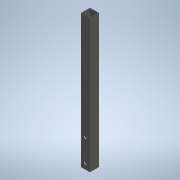
# Autodesk Inventor part: Carbon Fiber Arm
Saved by Autodesk Inventor 2021 (Build 250183000, 183)
## iProperties
Created: 2020-04-12
Part Number: Carbon Fiber Arm
Material: Generic
Document SubType Name: Modeling
Designer: chutsu
Density: 1 g/cm^3
Appearance: Default
Author: chutsu
Autodesk Inventor part; units mm, degrees
ref_plane "YZ Plane" through (0, 0, 0) normal (1, 0, 0) x (0, 1, 0)
ref_plane "XZ Plane" through (0, 0, 0) normal (0, 1, 0) x (-1, 0, 0)
ref_plane "XY Plane" through (0, 0, 0) normal (0, 0, 1) x (1, 0, 0)
sketch "Sketch1" plane through (0, 0, 0) normal (0, 1, 0) x (-1, 0, 0)
  line L0 (4, -4) -> (-4, -4)
  line L1 (-4, -4) -> (-4, 4)
  line L2 (-4, 4) -> (4, 4)
  line L3 (4, 4) -> (4, -4)
  line L4 (3.5, -3.5) -> (-3.5, -3.5)
  line L5 (-3.5, -3.5) -> (-3.5, 3.5)
  line L6 (-3.5, 3.5) -> (3.5, 3.5)
  line L7 (3.5, 3.5) -> (3.5, -3.5)
  line L8 (3.5, 0) -> (-3.5, 0)
  line L9 (0, -3.5) -> (0, 3.5)
  point P0 (0, 0)
  dimension "d0" = 0.5
  dimension "d1" = 0.5
  dimension "d2" = 0.5
  dimension "d3" = 0.5
  dimension "d4" = 7
  dimension "d5" = 7
  constraints: 20 end point, 6 midpoint, 4 parallel, 2 horizontal, 2 perpendicular
  measures "d0" distance between parallel lines of L7 L3
  measures "d1" distance between parallel lines of L1 L5
  measures "d2" distance between parallel lines of L0 L4
  measures "d3" distance between parallel lines of L2 L6
  measures "d4" distance between parallel lines of L5 L7
  measures "d5" distance between parallel lines of L6 L4
extrude "Extrusion1" add sketch "Sketch1" along normal blind 120
sketch "Sketch2" plane through (-4, 0, 4) normal (0, 0, 1) x (1, 0, 0)
  line L0 (4, 0) -> (4, 120)
  line L1 (0, 120) -> (8, 120) projected
  line L2 (0, 0) -> (8, 0) projected
  point P0 (4, 5)
  point P1 (4, 25)
  dimension "d8" = 20
  dimension "d9" = 5
  constraints: 2 end point, 2 point on line, 1 midpoint
  measures "d8" distance of point (4, 25) point (4, 5)
  measures "d9" distance from line of L2 point (4, 5)
hole "Hole1" at (0, 5, 4) at (0, 25, 4) direction (0, 0, -1) diameter 2.3 end through all
body "Solid1"
